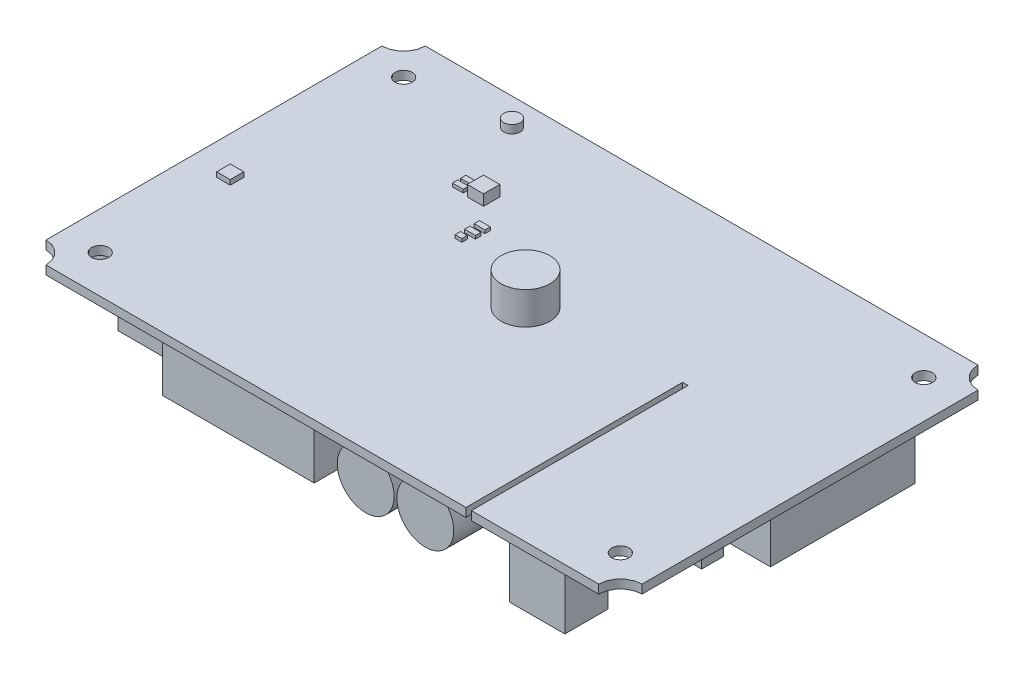
GridUp-PCB (Autodesk Fusion 360 design; units mm, degrees)
part number: 2026-09-14-08-15-55-205
Autodesk Fusion 360 part; units mm, degrees
sketch "Çizim1" plane through (0, 0, 0) normal (0, 0, 1) x (1, 0, 0)
  line L0 (0, 0) -> (110, 0)
  line L1 (110, 0) -> (110, 70)
  line L2 (110, 70) -> (0, 70)
  line L3 (0, 70) -> (0, 0)
sketch "Çizim2" plane through (0, 0, 0) normal (0, 0, 1) x (1, 0, 0)
  circle A0 centre (3.5, 3.5) radius 1.6
  circle A1 centre (106.5, 3.5) radius 1.6
  circle A2 centre (3.5, 66.5) radius 1.6
  circle A3 centre (106.5, 66.5) radius 1.6
  line L0 (81.5, -1) -> (82.5, -1)
  line L1 (82.5, -1) -> (82.5, 40)
  line L2 (82.5, 40) -> (81.5, 40)
  line L3 (81.5, 40) -> (81.5, -1)
ref_plane "WorkPlane1" through (0, 0, 1.6) normal (0, 0, 1) x (1, 0, 0)
sketch "Çizim3" plane through (0, 0, 1.6) normal (0, 0, 1) x (1, 0, 0)
  circle A0 centre (55, 37.5) radius 4.5
ref_plane "WorkPlane2" through (0, 0, 1.6) normal (0, 0, 1) x (1, 0, 0)
sketch "Çizim4" plane through (0, 0, 1.6) normal (0, 0, 1) x (1, 0, 0)
  line L0 (5.75, 29.75) -> (8.25, 29.75)
  line L1 (8.25, 29.75) -> (8.25, 32.25)
  line L2 (8.25, 32.25) -> (5.75, 32.25)
  line L3 (5.75, 32.25) -> (5.75, 29.75)
ref_plane "WorkPlane3" through (0, 0, 1.6) normal (0, 0, 1) x (1, 0, 0)
sketch "Çizim5" plane through (0, 0, 1.6) normal (0, 0, 1) x (1, 0, 0)
  circle A0 centre (25, 65) radius 1.5
ref_plane "WorkPlane4" through (0, 0, 1.6) normal (0, 0, 1) x (1, 0, 0)
sketch "Çizim6" plane through (0, 0, 1.6) normal (0, 0, 1) x (1, 0, 0)
  line L0 (37.5, 45.5) -> (39.5, 45.5)
  line L1 (39.5, 45.5) -> (39.5, 46.5)
  line L2 (39.5, 46.5) -> (37.5, 46.5)
  line L3 (37.5, 46.5) -> (37.5, 45.5)
ref_plane "WorkPlane5" through (0, 0, 1.6) normal (0, 0, 1) x (1, 0, 0)
sketch "Çizim7" plane through (0, 0, 1.6) normal (0, 0, 1) x (1, 0, 0)
  line L0 (37.5, 43.75) -> (39.5, 43.75)
  line L1 (39.5, 43.75) -> (39.5, 44.75)
  line L2 (39.5, 44.75) -> (37.5, 44.75)
  line L3 (37.5, 44.75) -> (37.5, 43.75)
ref_plane "WorkPlane6" through (0, 0, 1.6) normal (0, 0, 1) x (1, 0, 0)
sketch "Çizim8" plane through (0, 0, 1.6) normal (0, 0, 1) x (1, 0, 0)
  line L0 (37.5, 42) -> (38.75, 42)
  line L1 (38.75, 42) -> (38.75, 43)
  line L2 (38.75, 43) -> (37.5, 43)
  line L3 (37.5, 43) -> (37.5, 42)
ref_plane "WorkPlane7" through (0, 0, 1.6) normal (0, 0, 1) x (1, 0, 0)
sketch "Çizim9" plane through (0, 0, 1.6) normal (0, 0, 1) x (1, 0, 0)
  line L0 (27, 51.5) -> (29, 51.5)
  line L1 (29, 51.5) -> (29, 52.5)
  line L2 (29, 52.5) -> (27, 52.5)
  line L3 (27, 52.5) -> (27, 51.5)
ref_plane "WorkPlane8" through (0, 0, 1.6) normal (0, 0, 1) x (1, 0, 0)
sketch "Çizim10" plane through (0, 0, 1.6) normal (0, 0, 1) x (1, 0, 0)
  line L0 (27, 50) -> (29, 50)
  line L1 (29, 50) -> (29, 51)
  line L2 (29, 51) -> (27, 51)
  line L3 (27, 51) -> (27, 50)
ref_plane "WorkPlane9" through (0, 0, 1.6) normal (0, 0, 1) x (1, 0, 0)
sketch "Çizim11" plane through (0, 0, 1.6) normal (0, 0, 1) x (1, 0, 0)
  line L0 (30, 49.75) -> (33, 49.75)
  line L1 (33, 49.75) -> (33, 52.75)
  line L2 (33, 52.75) -> (30, 52.75)
  line L3 (30, 52.75) -> (30, 49.75)
ref_plane "WorkPlane10" through (0, 0, 0) normal (0, 0, 1) x (1, 0, 0)
sketch "Çizim12" plane through (0, 0, 0) normal (0, 0, 1) x (1, 0, 0)
  line L0 (6, 44.8) -> (24, 44.8)
  line L1 (24, 44.8) -> (24, 64)
  line L2 (24, 64) -> (6, 64)
  line L3 (6, 64) -> (6, 44.8)
ref_plane "WorkPlane11" through (0, 0, 0) normal (0, 0, 1) x (1, 0, 0)
sketch "Çizim13" plane through (0, 0, 0) normal (0, 0, 1) x (1, 0, 0)
  line L0 (66, 43.75) -> (99.8, 43.75)
  line L1 (99.8, 43.75) -> (99.8, 64.05)
  line L2 (99.8, 64.05) -> (66, 64.05)
  line L3 (66, 64.05) -> (66, 43.75)
ref_plane "WorkPlane12" through (0, 0, 0) normal (0, 0, 1) x (1, 0, 0)
sketch "Çizim14" plane through (0, 0, 0) normal (0, 0, 1) x (1, 0, 0)
  line L0 (88, 22.25) -> (94.1, 22.25)
  line L1 (94.1, 22.25) -> (94.1, 25)
  line L2 (94.1, 25) -> (88, 25)
  line L3 (88, 25) -> (88, 22.25)
ref_plane "WorkPlane13" through (0, 0, 0) normal (0, 0, 1) x (1, 0, 0)
sketch "Çizim15" plane through (0, 0, 0) normal (0, 0, 1) x (1, 0, 0)
  line L0 (96.5, 21.5) -> (103.5, 21.5)
  line L1 (103.5, 21.5) -> (103.5, 25.5)
  line L2 (103.5, 25.5) -> (96.5, 25.5)
  line L3 (96.5, 25.5) -> (96.5, 21.5)
ref_plane "WorkPlane14" through (0, 0, 0) normal (0, 0, 1) x (1, 0, 0)
sketch "Çizim16" plane through (0, 0, 0) normal (0, 0, 1) x (1, 0, 0)
  line L0 (92, 0.5) -> (102.25, 0.5)
  line L1 (102.25, 0.5) -> (102.25, 8.5)
  line L2 (102.25, 8.5) -> (92, 8.5)
  line L3 (92, 8.5) -> (92, 0.5)
ref_plane "WorkPlane15" through (0, 0, 0) normal (0, 0, 1) x (1, 0, 0)
sketch "Çizim17" plane through (0, 0, 0) normal (0, 0, 1) x (1, 0, 0)
  line L0 (70, 35) -> (76.5, 35)
  line L1 (76.5, 35) -> (76.5, 42)
  line L2 (76.5, 42) -> (70, 42)
  line L3 (70, 42) -> (70, 35)
ref_plane "WorkPlane16" through (0, 0, 0) normal (0, 0, 1) x (1, 0, 0)
sketch "Çizim18" plane through (0, 0, 0) normal (0, 0, 1) x (1, 0, 0)
  line L0 (76.75, 39.1) -> (81, 39.1)
  line L1 (81, 39.1) -> (81, 41.75)
  line L2 (81, 41.75) -> (76.75, 41.75)
  line L3 (76.75, 41.75) -> (76.75, 39.1)
ref_plane "WorkPlane17" through (0, 0, 0) normal (0, 0, 1) x (1, 0, 0)
sketch "Çizim19" plane through (0, 0, 0) normal (0, 0, 1) x (1, 0, 0)
  line L0 (76.75, 35.1) -> (81, 35.1)
  line L1 (81, 35.1) -> (81, 37.75)
  line L2 (81, 37.75) -> (76.75, 37.75)
  line L3 (76.75, 37.75) -> (76.75, 35.1)
ref_plane "WorkPlane18" through (0, 0, 0) normal (0, 0, 1) x (1, 0, 0)
sketch "Çizim20" plane through (0, 0, 0) normal (0, 0, 1) x (1, 0, 0)
  line L0 (75, 44.5) -> (77, 44.5)
  line L1 (77, 44.5) -> (77, 45.5)
  line L2 (77, 45.5) -> (75, 45.5)
  line L3 (75, 45.5) -> (75, 44.5)
ref_plane "WorkPlane19" through (0, 0, 0) normal (0, 0, 1) x (1, 0, 0)
sketch "Çizim21" plane through (0, 0, 0) normal (0, 0, 1) x (1, 0, 0)
  line L0 (75, 29.5) -> (77, 29.5)
  line L1 (77, 29.5) -> (77, 30.5)
  line L2 (77, 30.5) -> (75, 30.5)
  line L3 (75, 30.5) -> (75, 29.5)
ref_plane "WorkPlane20" through (0, 0, 0) normal (0, 0, 1) x (1, 0, 0)
sketch "Çizim22" plane through (0, 0, 0) normal (0, 0, 1) x (1, 0, 0)
  line L0 (75, 28) -> (77, 28)
  line L1 (77, 28) -> (77, 29)
  line L2 (77, 29) -> (75, 29)
  line L3 (75, 29) -> (75, 28)
ref_plane "WorkPlane21" through (0, 13.75, 0) normal (0, 1, 0) x (0, 0, 1)
sketch "Çizim23" plane through (0, 13.75, 0) normal (0, 1, 0) x (1, 0, 0)
  circle A0 centre (65.75, 10.75) radius 10.75
ref_plane "WorkPlane22" through (0, 0, 0) normal (0, 0, 1) x (1, 0, 0)
sketch "Çizim24" plane through (0, 0, 0) normal (0, 0, 1) x (1, 0, 0)
  line L0 (41.25, 14) -> (46.25, 14)
  line L1 (46.25, 14) -> (46.25, 20)
  line L2 (46.25, 20) -> (41.25, 20)
  line L3 (41.25, 20) -> (41.25, 14)
ref_plane "WorkPlane23" through (0, 0, 0) normal (0, 0, 1) x (1, 0, 0)
sketch "Çizim25" plane through (0, 0, 0) normal (0, 0, 1) x (1, 0, 0)
  line L0 (47.5, 15) -> (48.5, 15)
  line L1 (48.5, 15) -> (48.5, 17)
  line L2 (48.5, 17) -> (47.5, 17)
  line L3 (47.5, 17) -> (47.5, 15)
ref_plane "WorkPlane24" through (0, 0, 0) normal (0, 0, 1) x (1, 0, 0)
sketch "Çizim26" plane through (0, 0, 0) normal (0, 0, 1) x (1, 0, 0)
  line L0 (1, 6.25) -> (9, 6.25)
  line L1 (9, 6.25) -> (9, 21.5)
  line L2 (9, 21.5) -> (1, 21.5)
  line L3 (1, 21.5) -> (1, 6.25)
ref_plane "WorkPlane25" through (0, 0, 0) normal (0, 0, 1) x (1, 0, 0)
sketch "Çizim27" plane through (0, 0, 0) normal (0, 0, 1) x (1, 0, 0)
  line L0 (25, 14) -> (27, 14)
  line L1 (27, 14) -> (27, 15)
  line L2 (27, 15) -> (25, 15)
  line L3 (25, 15) -> (25, 14)
ref_plane "WorkPlane26" through (0, 0, 0) normal (0, 0, 1) x (1, 0, 0)
sketch "Çizim28" plane through (0, 0, 0) normal (0, 0, 1) x (1, 0, 0)
  line L0 (28, 14) -> (30, 14)
  line L1 (30, 14) -> (30, 15)
  line L2 (30, 15) -> (28, 15)
  line L3 (28, 15) -> (28, 14)
ref_plane "WorkPlane27" through (0, 0, 0) normal (0, 0, 1) x (1, 0, 0)
sketch "Çizim29" plane through (0, 0, 0) normal (0, 0, 1) x (1, 0, 0)
  line L0 (31, 14) -> (33, 14)
  line L1 (33, 14) -> (33, 15)
  line L2 (33, 15) -> (31, 15)
  line L3 (31, 15) -> (31, 14)
ref_plane "WorkPlane28" through (0, 0, 0) normal (0, 0, 1) x (1, 0, 0)
sketch "Çizim30" plane through (0, 0, 0) normal (0, 0, 1) x (1, 0, 0)
  line L0 (34, 14) -> (36, 14)
  line L1 (36, 14) -> (36, 15)
  line L2 (36, 15) -> (34, 15)
  line L3 (34, 15) -> (34, 14)
ref_plane "WorkPlane29" through (0, 0, 0) normal (0, 0, 1) x (1, 0, 0)
sketch "Çizim31" plane through (0, 0, 0) normal (0, 0, 1) x (1, 0, 0)
  line L0 (37, 13) -> (39, 13)
  line L1 (39, 13) -> (39, 15)
  line L2 (39, 15) -> (37, 15)
  line L3 (37, 15) -> (37, 13)
ref_plane "WorkPlane30" through (0, 0, 0) normal (0, 0, 1) x (1, 0, 0)
sketch "Çizim32" plane through (0, 0, 0) normal (0, 0, 1) x (1, 0, 0)
  line L0 (25, 0.5) -> (53, 0.5)
  line L1 (53, 0.5) -> (53, 7.5)
  line L2 (53, 7.5) -> (25, 7.5)
  line L3 (25, 7.5) -> (25, 0.5)
ref_plane "WorkPlane31" through (0, 0, 0) normal (0, 0, 1) x (1, 0, 0)
sketch "Çizim33" plane through (0, 0, 0) normal (0, 0, 1) x (1, 0, 0)
  line L0 (11, 6.25) -> (24, 6.25)
  line L1 (24, 6.25) -> (24, 11.25)
  line L2 (24, 11.25) -> (11, 11.25)
  line L3 (11, 11.25) -> (11, 6.25)
sketch "Çizim34" plane through (0, 0, 0) normal (0, 0, 1) x (1, 0, 0)
  line L0 (0, 0) -> (110, 0)
  line L1 (110, 0) -> (110, 70)
  line L2 (110, 70) -> (0, 70)
  line L3 (0, 70) -> (0, 0)
sketch "Çizim35" plane through (0, 0, 0) normal (0, 0, 1) x (1, 0, 0)
  circle A0 centre (7, 7) radius 1.6
  circle A1 centre (103, 7) radius 1.6
  circle A2 centre (7, 63) radius 1.6
  circle A3 centre (103, 63) radius 1.6
  line L0 (81.5, -1) -> (82.5, -1)
  line L1 (82.5, -1) -> (82.5, 40)
  line L2 (82.5, 40) -> (81.5, 40)
  line L3 (81.5, 40) -> (81.5, -1)
  circle A4 centre (0, 0) radius 4
  circle A5 centre (110, 0) radius 4
  circle A6 centre (0, 70) radius 4
  circle A7 centre (110, 70) radius 4
ref_plane "WorkPlane32" through (0, 0, 1.6) normal (0, 0, 1) x (1, 0, 0)
sketch "Çizim36" plane through (0, 0, 1.6) normal (0, 0, 1) x (1, 0, 0)
  circle A0 centre (55, 37.5) radius 4.5
ref_plane "WorkPlane33" through (0, 0, 1.6) normal (0, 0, 1) x (1, 0, 0)
sketch "Çizim37" plane through (0, 0, 1.6) normal (0, 0, 1) x (1, 0, 0)
  line L0 (5.75, 29.75) -> (8.25, 29.75)
  line L1 (8.25, 29.75) -> (8.25, 32.25)
  line L2 (8.25, 32.25) -> (5.75, 32.25)
  line L3 (5.75, 32.25) -> (5.75, 29.75)
ref_plane "WorkPlane34" through (0, 0, 1.6) normal (0, 0, 1) x (1, 0, 0)
sketch "Çizim38" plane through (0, 0, 1.6) normal (0, 0, 1) x (1, 0, 0)
  circle A0 centre (25, 65) radius 1.5
ref_plane "WorkPlane35" through (0, 0, 1.6) normal (0, 0, 1) x (1, 0, 0)
sketch "Çizim39" plane through (0, 0, 1.6) normal (0, 0, 1) x (1, 0, 0)
  line L0 (37.5, 45.5) -> (39.5, 45.5)
  line L1 (39.5, 45.5) -> (39.5, 46.5)
  line L2 (39.5, 46.5) -> (37.5, 46.5)
  line L3 (37.5, 46.5) -> (37.5, 45.5)
ref_plane "WorkPlane36" through (0, 0, 1.6) normal (0, 0, 1) x (1, 0, 0)
sketch "Çizim40" plane through (0, 0, 1.6) normal (0, 0, 1) x (1, 0, 0)
  line L0 (37.5, 43.75) -> (39.5, 43.75)
  line L1 (39.5, 43.75) -> (39.5, 44.75)
  line L2 (39.5, 44.75) -> (37.5, 44.75)
  line L3 (37.5, 44.75) -> (37.5, 43.75)
ref_plane "WorkPlane37" through (0, 0, 1.6) normal (0, 0, 1) x (1, 0, 0)
sketch "Çizim41" plane through (0, 0, 1.6) normal (0, 0, 1) x (1, 0, 0)
  line L0 (37.5, 42) -> (38.75, 42)
  line L1 (38.75, 42) -> (38.75, 43)
  line L2 (38.75, 43) -> (37.5, 43)
  line L3 (37.5, 43) -> (37.5, 42)
ref_plane "WorkPlane38" through (0, 0, 1.6) normal (0, 0, 1) x (1, 0, 0)
sketch "Çizim42" plane through (0, 0, 1.6) normal (0, 0, 1) x (1, 0, 0)
  line L0 (29, 51.5) -> (31, 51.5)
  line L1 (31, 51.5) -> (31, 52.5)
  line L2 (31, 52.5) -> (29, 52.5)
  line L3 (29, 52.5) -> (29, 51.5)
ref_plane "WorkPlane39" through (0, 0, 1.6) normal (0, 0, 1) x (1, 0, 0)
sketch "Çizim43" plane through (0, 0, 1.6) normal (0, 0, 1) x (1, 0, 0)
  line L0 (29, 50) -> (31, 50)
  line L1 (31, 50) -> (31, 51)
  line L2 (31, 51) -> (29, 51)
  line L3 (29, 51) -> (29, 50)
ref_plane "WorkPlane40" through (0, 0, 1.6) normal (0, 0, 1) x (1, 0, 0)
sketch "Çizim44" plane through (0, 0, 1.6) normal (0, 0, 1) x (1, 0, 0)
  line L0 (32, 49.75) -> (35, 49.75)
  line L1 (35, 49.75) -> (35, 52.75)
  line L2 (35, 52.75) -> (32, 52.75)
  line L3 (32, 52.75) -> (32, 49.75)
ref_plane "WorkPlane41" through (0, 0, 0) normal (0, 0, 1) x (1, 0, 0)
sketch "Çizim45" plane through (0, 0, 0) normal (0, 0, 1) x (1, 0, 0)
  line L0 (10, 40.8) -> (28, 40.8)
  line L1 (28, 40.8) -> (28, 60)
  line L2 (28, 60) -> (10, 60)
  line L3 (10, 60) -> (10, 40.8)
ref_plane "WorkPlane42" through (0, 0, 0) normal (0, 0, 1) x (1, 0, 0)
sketch "Çizim46" plane through (0, 0, 0) normal (0, 0, 1) x (1, 0, 0)
  line L0 (64, 43.75) -> (97.8, 43.75)
  line L1 (97.8, 43.75) -> (97.8, 64.05)
  line L2 (97.8, 64.05) -> (64, 64.05)
  line L3 (64, 64.05) -> (64, 43.75)
ref_plane "WorkPlane43" through (0, 0, 0) normal (0, 0, 1) x (1, 0, 0)
sketch "Çizim47" plane through (0, 0, 0) normal (0, 0, 1) x (1, 0, 0)
  line L0 (88, 22.25) -> (94.1, 22.25)
  line L1 (94.1, 22.25) -> (94.1, 25)
  line L2 (94.1, 25) -> (88, 25)
  line L3 (88, 25) -> (88, 22.25)
ref_plane "WorkPlane44" through (0, 0, 0) normal (0, 0, 1) x (1, 0, 0)
sketch "Çizim48" plane through (0, 0, 0) normal (0, 0, 1) x (1, 0, 0)
  line L0 (96.5, 21.5) -> (103.5, 21.5)
  line L1 (103.5, 21.5) -> (103.5, 25.5)
  line L2 (103.5, 25.5) -> (96.5, 25.5)
  line L3 (96.5, 25.5) -> (96.5, 21.5)
ref_plane "WorkPlane45" through (0, 0, 0) normal (0, 0, 1) x (1, 0, 0)
sketch "Çizim49" plane through (0, 0, 0) normal (0, 0, 1) x (1, 0, 0)
  line L0 (89, 0.5) -> (99.25, 0.5)
  line L1 (99.25, 0.5) -> (99.25, 8.5)
  line L2 (99.25, 8.5) -> (89, 8.5)
  line L3 (89, 8.5) -> (89, 0.5)
ref_plane "WorkPlane46" through (0, 0, 0) normal (0, 0, 1) x (1, 0, 0)
sketch "Çizim50" plane through (0, 0, 0) normal (0, 0, 1) x (1, 0, 0)
  line L0 (70, 35) -> (76.5, 35)
  line L1 (76.5, 35) -> (76.5, 42)
  line L2 (76.5, 42) -> (70, 42)
  line L3 (70, 42) -> (70, 35)
ref_plane "WorkPlane47" through (0, 0, 0) normal (0, 0, 1) x (1, 0, 0)
sketch "Çizim51" plane through (0, 0, 0) normal (0, 0, 1) x (1, 0, 0)
  line L0 (76.75, 39.1) -> (81, 39.1)
  line L1 (81, 39.1) -> (81, 41.75)
  line L2 (81, 41.75) -> (76.75, 41.75)
  line L3 (76.75, 41.75) -> (76.75, 39.1)
ref_plane "WorkPlane48" through (0, 0, 0) normal (0, 0, 1) x (1, 0, 0)
sketch "Çizim52" plane through (0, 0, 0) normal (0, 0, 1) x (1, 0, 0)
  line L0 (76.75, 35.1) -> (81, 35.1)
  line L1 (81, 35.1) -> (81, 37.75)
  line L2 (81, 37.75) -> (76.75, 37.75)
  line L3 (76.75, 37.75) -> (76.75, 35.1)
ref_plane "WorkPlane49" through (0, 0, 0) normal (0, 0, 1) x (1, 0, 0)
sketch "Çizim53" plane through (0, 0, 0) normal (0, 0, 1) x (1, 0, 0)
  line L0 (60.5, 44.5) -> (62.5, 44.5)
  line L1 (62.5, 44.5) -> (62.5, 45.5)
  line L2 (62.5, 45.5) -> (60.5, 45.5)
  line L3 (60.5, 45.5) -> (60.5, 44.5)
ref_plane "WorkPlane50" through (0, 0, 0) normal (0, 0, 1) x (1, 0, 0)
sketch "Çizim54" plane through (0, 0, 0) normal (0, 0, 1) x (1, 0, 0)
  line L0 (75, 29.5) -> (77, 29.5)
  line L1 (77, 29.5) -> (77, 30.5)
  line L2 (77, 30.5) -> (75, 30.5)
  line L3 (75, 30.5) -> (75, 29.5)
ref_plane "WorkPlane51" through (0, 0, 0) normal (0, 0, 1) x (1, 0, 0)
sketch "Çizim55" plane through (0, 0, 0) normal (0, 0, 1) x (1, 0, 0)
  line L0 (75, 28) -> (77, 28)
  line L1 (77, 28) -> (77, 29)
  line L2 (77, 29) -> (75, 29)
  line L3 (75, 29) -> (75, 28)
ref_plane "WorkPlane52" through (0, 13.75, 0) normal (0, 1, 0) x (0, 0, 1)
sketch "Çizim56" plane through (0, 13.75, 0) normal (0, 1, 0) x (1, 0, 0)
  circle A0 centre (65.75, 10.75) radius 10.75
ref_plane "WorkPlane53" through (0, 0, 0) normal (0, 0, 1) x (1, 0, 0)
sketch "Çizim57" plane through (0, 0, 0) normal (0, 0, 1) x (1, 0, 0)
  line L0 (41.25, 14) -> (46.25, 14)
  line L1 (46.25, 14) -> (46.25, 20)
  line L2 (46.25, 20) -> (41.25, 20)
  line L3 (41.25, 20) -> (41.25, 14)
ref_plane "WorkPlane54" through (0, 0, 0) normal (0, 0, 1) x (1, 0, 0)
sketch "Çizim58" plane through (0, 0, 0) normal (0, 0, 1) x (1, 0, 0)
  line L0 (47.5, 15) -> (48.5, 15)
  line L1 (48.5, 15) -> (48.5, 17)
  line L2 (48.5, 17) -> (47.5, 17)
  line L3 (47.5, 17) -> (47.5, 15)
ref_plane "WorkPlane55" through (0, 0, 0) normal (0, 0, 1) x (1, 0, 0)
sketch "Çizim59" plane through (0, 0, 0) normal (0, 0, 1) x (1, 0, 0)
  line L0 (1, 11) -> (9, 11)
  line L1 (9, 11) -> (9, 26.25)
  line L2 (9, 26.25) -> (1, 26.25)
  line L3 (1, 26.25) -> (1, 11)
ref_plane "WorkPlane56" through (0, 0, 0) normal (0, 0, 1) x (1, 0, 0)
sketch "Çizim60" plane through (0, 0, 0) normal (0, 0, 1) x (1, 0, 0)
  line L0 (25, 14) -> (27, 14)
  line L1 (27, 14) -> (27, 15)
  line L2 (27, 15) -> (25, 15)
  line L3 (25, 15) -> (25, 14)
ref_plane "WorkPlane57" through (0, 0, 0) normal (0, 0, 1) x (1, 0, 0)
sketch "Çizim61" plane through (0, 0, 0) normal (0, 0, 1) x (1, 0, 0)
  line L0 (28, 14) -> (30, 14)
  line L1 (30, 14) -> (30, 15)
  line L2 (30, 15) -> (28, 15)
  line L3 (28, 15) -> (28, 14)
ref_plane "WorkPlane58" through (0, 0, 0) normal (0, 0, 1) x (1, 0, 0)
sketch "Çizim62" plane through (0, 0, 0) normal (0, 0, 1) x (1, 0, 0)
  line L0 (31, 14) -> (33, 14)
  line L1 (33, 14) -> (33, 15)
  line L2 (33, 15) -> (31, 15)
  line L3 (31, 15) -> (31, 14)
ref_plane "WorkPlane59" through (0, 0, 0) normal (0, 0, 1) x (1, 0, 0)
sketch "Çizim63" plane through (0, 0, 0) normal (0, 0, 1) x (1, 0, 0)
  line L0 (34, 14) -> (36, 14)
  line L1 (36, 14) -> (36, 15)
  line L2 (36, 15) -> (34, 15)
  line L3 (34, 15) -> (34, 14)
ref_plane "WorkPlane60" through (0, 0, 0) normal (0, 0, 1) x (1, 0, 0)
sketch "Çizim64" plane through (0, 0, 0) normal (0, 0, 1) x (1, 0, 0)
  line L0 (37, 13) -> (39, 13)
  line L1 (39, 13) -> (39, 15)
  line L2 (39, 15) -> (37, 15)
  line L3 (37, 15) -> (37, 13)
ref_plane "WorkPlane61" through (0, 0, 0) normal (0, 0, 1) x (1, 0, 0)
sketch "Çizim65" plane through (0, 0, 0) normal (0, 0, 1) x (1, 0, 0)
  line L0 (25, 0.5) -> (53, 0.5)
  line L1 (53, 0.5) -> (53, 7.5)
  line L2 (53, 7.5) -> (25, 7.5)
  line L3 (25, 7.5) -> (25, 0.5)
ref_plane "WorkPlane62" through (0, 0, 0) normal (0, 0, 1) x (1, 0, 0)
sketch "Çizim66" plane through (0, 0, 0) normal (0, 0, 1) x (1, 0, 0)
  line L0 (11, 6.25) -> (24, 6.25)
  line L1 (24, 6.25) -> (24, 11.25)
  line L2 (24, 11.25) -> (11, 11.25)
  line L3 (11, 11.25) -> (11, 6.25)
sketch "Çizim67" plane through (0, 0, 0) normal (0, 0, 1) x (1, 0, 0)
  line L0 (0, 0) -> (110, 0)
  line L1 (110, 0) -> (110, 70)
  line L2 (110, 70) -> (0, 70)
  line L3 (0, 70) -> (0, 0)
extrude "Ekstrüzyon67" add sketch "Çizim67" along normal blind 1.6 makes body 1
fillet "Radyus3" radius 2 4 edges at (0, 70, 0.8) (110, 70, 0.8) (110, 0, 0.8) (0, 0, 0.8) on bodies 1
sketch "Çizim68" plane through (0, 0, 0) normal (0, 0, 1) x (1, 0, 0)
  circle A0 centre (7, 7) radius 1.6
  circle A1 centre (103, 7) radius 1.6
  circle A2 centre (7, 63) radius 1.6
  circle A3 centre (103, 63) radius 1.6
  line L0 (81.5, -1) -> (82.5, -1)
  line L1 (82.5, -1) -> (82.5, 40)
  line L2 (82.5, 40) -> (81.5, 40)
  line L3 (81.5, 40) -> (81.5, -1)
  circle A4 centre (0, 0) radius 4
  circle A5 centre (110, 0) radius 4
  circle A6 centre (0, 70) radius 4
  circle A7 centre (110, 70) radius 4
extrude "Ekstrüzyon68" cut sketch "Çizim68" along normal mid plane 10 bodies 1
ref_plane "WorkPlane63" through (0, 0, 1.6) normal (0, 0, 1) x (1, 0, 0)
sketch "Çizim69" plane through (0, 0, 1.6) normal (0, 0, 1) x (1, 0, 0)
  circle A0 centre (55, 37.5) radius 4.5
extrude "Ekstrüzyon69" add sketch "Çizim69" along normal blind 6 separate body makes body 2
ref_plane "WorkPlane64" through (0, 0, 1.6) normal (0, 0, 1) x (1, 0, 0)
sketch "Çizim70" plane through (0, 0, 1.6) normal (0, 0, 1) x (1, 0, 0)
  line L0 (5.75, 29.75) -> (8.25, 29.75)
  line L1 (8.25, 29.75) -> (8.25, 32.25)
  line L2 (8.25, 32.25) -> (5.75, 32.25)
  line L3 (5.75, 32.25) -> (5.75, 29.75)
extrude "Ekstrüzyon70" add sketch "Çizim70" along normal blind 0.9 separate body makes body 3
ref_plane "WorkPlane65" through (0, 0, 1.6) normal (0, 0, 1) x (1, 0, 0)
sketch "Çizim71" plane through (0, 0, 1.6) normal (0, 0, 1) x (1, 0, 0)
  circle A0 centre (25, 65) radius 1.5
extrude "Ekstrüzyon71" add sketch "Çizim71" along normal blind 1.5 separate body makes body 4
ref_plane "WorkPlane66" through (0, 0, 1.6) normal (0, 0, 1) x (1, 0, 0)
sketch "Çizim72" plane through (0, 0, 1.6) normal (0, 0, 1) x (1, 0, 0)
  line L0 (37.5, 45.5) -> (39.5, 45.5)
  line L1 (39.5, 45.5) -> (39.5, 46.5)
  line L2 (39.5, 46.5) -> (37.5, 46.5)
  line L3 (37.5, 46.5) -> (37.5, 45.5)
extrude "Ekstrüzyon72" add sketch "Çizim72" along normal blind 0.6 separate body makes body 5
ref_plane "WorkPlane67" through (0, 0, 1.6) normal (0, 0, 1) x (1, 0, 0)
sketch "Çizim73" plane through (0, 0, 1.6) normal (0, 0, 1) x (1, 0, 0)
  line L0 (37.5, 43.75) -> (39.5, 43.75)
  line L1 (39.5, 43.75) -> (39.5, 44.75)
  line L2 (39.5, 44.75) -> (37.5, 44.75)
  line L3 (37.5, 44.75) -> (37.5, 43.75)
extrude "Ekstrüzyon73" add sketch "Çizim73" along normal blind 0.6 separate body makes body 6
ref_plane "WorkPlane68" through (0, 0, 1.6) normal (0, 0, 1) x (1, 0, 0)
sketch "Çizim74" plane through (0, 0, 1.6) normal (0, 0, 1) x (1, 0, 0)
  line L0 (37.5, 42) -> (38.75, 42)
  line L1 (38.75, 42) -> (38.75, 43)
  line L2 (38.75, 43) -> (37.5, 43)
  line L3 (37.5, 43) -> (37.5, 42)
extrude "Ekstrüzyon74" add sketch "Çizim74" along normal blind 0.6 separate body makes body 7
ref_plane "WorkPlane69" through (0, 0, 1.6) normal (0, 0, 1) x (1, 0, 0)
sketch "Çizim75" plane through (0, 0, 1.6) normal (0, 0, 1) x (1, 0, 0)
  line L0 (29, 51.5) -> (31, 51.5)
  line L1 (31, 51.5) -> (31, 52.5)
  line L2 (31, 52.5) -> (29, 52.5)
  line L3 (29, 52.5) -> (29, 51.5)
extrude "Ekstrüzyon75" add sketch "Çizim75" along normal blind 0.6 separate body makes body 8
ref_plane "WorkPlane70" through (0, 0, 1.6) normal (0, 0, 1) x (1, 0, 0)
sketch "Çizim76" plane through (0, 0, 1.6) normal (0, 0, 1) x (1, 0, 0)
  line L0 (29, 50) -> (31, 50)
  line L1 (31, 50) -> (31, 51)
  line L2 (31, 51) -> (29, 51)
  line L3 (29, 51) -> (29, 50)
extrude "Ekstrüzyon76" add sketch "Çizim76" along normal blind 0.6 separate body makes body 9
ref_plane "WorkPlane71" through (0, 0, 1.6) normal (0, 0, 1) x (1, 0, 0)
sketch "Çizim77" plane through (0, 0, 1.6) normal (0, 0, 1) x (1, 0, 0)
  line L0 (32, 49.75) -> (35, 49.75)
  line L1 (35, 49.75) -> (35, 52.75)
  line L2 (35, 52.75) -> (32, 52.75)
  line L3 (32, 52.75) -> (32, 49.75)
extrude "Ekstrüzyon77" add sketch "Çizim77" along normal blind 2 separate body makes body 10
ref_plane "WorkPlane72" through (0, 0, 0) normal (0, 0, 1) x (1, 0, 0)
sketch "Çizim78" plane through (0, 0, 0) normal (0, 0, 1) x (1, 0, 0)
  line L0 (10, 40.8) -> (28, 40.8)
  line L1 (28, 40.8) -> (28, 60)
  line L2 (28, 60) -> (10, 60)
  line L3 (10, 60) -> (10, 40.8)
extrude "Ekstrüzyon78" add sketch "Çizim78" against normal blind 3.2 separate body makes body 11
ref_plane "WorkPlane73" through (0, 0, 0) normal (0, 0, 1) x (1, 0, 0)
sketch "Çizim79" plane through (0, 0, 0) normal (0, 0, 1) x (1, 0, 0)
  line L0 (64, 42) -> (95.7, 42)
  line L1 (95.7, 42) -> (95.7, 68.7)
  line L2 (95.7, 68.7) -> (64, 68.7)
  line L3 (64, 68.7) -> (64, 42)
extrude "Ekstrüzyon79" add sketch "Çizim79" against normal blind 21.8 separate body makes body 12
ref_plane "WorkPlane74" through (0, 0, 0) normal (0, 0, 1) x (1, 0, 0)
sketch "Çizim80" plane through (0, 0, 0) normal (0, 0, 1) x (1, 0, 0)
  line L0 (88, 22.25) -> (94.1, 22.25)
  line L1 (94.1, 22.25) -> (94.1, 25)
  line L2 (94.1, 25) -> (88, 25)
  line L3 (88, 25) -> (88, 22.25)
extrude "Ekstrüzyon80" add sketch "Çizim80" against normal blind 2.6 separate body makes body 13
ref_plane "WorkPlane75" through (0, 0, 0) normal (0, 0, 1) x (1, 0, 0)
sketch "Çizim81" plane through (0, 0, 0) normal (0, 0, 1) x (1, 0, 0)
  line L0 (96.5, 21.5) -> (103.5, 21.5)
  line L1 (103.5, 21.5) -> (103.5, 25.5)
  line L2 (103.5, 25.5) -> (96.5, 25.5)
  line L3 (96.5, 25.5) -> (96.5, 21.5)
extrude "Ekstrüzyon81" add sketch "Çizim81" against normal blind 8 separate body makes body 14
ref_plane "WorkPlane76" through (0, 0, 0) normal (0, 0, 1) x (1, 0, 0)
sketch "Çizim82" plane through (0, 0, 0) normal (0, 0, 1) x (1, 0, 0)
  line L0 (89, 0.5) -> (99.25, 0.5)
  line L1 (99.25, 0.5) -> (99.25, 8.5)
  line L2 (99.25, 8.5) -> (89, 8.5)
  line L3 (89, 8.5) -> (89, 0.5)
extrude "Ekstrüzyon82" add sketch "Çizim82" against normal blind 10 separate body makes body 15
ref_plane "WorkPlane77" through (0, 0, 0) normal (0, 0, 1) x (1, 0, 0)
sketch "Çizim83" plane through (0, 0, 0) normal (0, 0, 1) x (1, 0, 0)
  line L0 (70, 34) -> (76.5, 34)
  line L1 (76.5, 34) -> (76.5, 41)
  line L2 (76.5, 41) -> (70, 41)
  line L3 (70, 41) -> (70, 34)
extrude "Ekstrüzyon83" add sketch "Çizim83" against normal blind 1.7 separate body makes body 16
ref_plane "WorkPlane78" through (0, 0, 0) normal (0, 0, 1) x (1, 0, 0)
sketch "Çizim84" plane through (0, 0, 0) normal (0, 0, 1) x (1, 0, 0)
  line L0 (76.75, 39) -> (81, 39)
  line L1 (81, 39) -> (81, 41.65)
  line L2 (81, 41.65) -> (76.75, 41.65)
  line L3 (76.75, 41.65) -> (76.75, 39)
extrude "Ekstrüzyon84" add sketch "Çizim84" against normal blind 1.5 separate body makes body 17
ref_plane "WorkPlane79" through (0, 0, 0) normal (0, 0, 1) x (1, 0, 0)
sketch "Çizim85" plane through (0, 0, 0) normal (0, 0, 1) x (1, 0, 0)
  line L0 (76.75, 35) -> (81, 35)
  line L1 (81, 35) -> (81, 37.65)
  line L2 (81, 37.65) -> (76.75, 37.65)
  line L3 (76.75, 37.65) -> (76.75, 35)
extrude "Ekstrüzyon85" add sketch "Çizim85" against normal blind 1.5 separate body makes body 18
ref_plane "WorkPlane80" through (0, 0, 0) normal (0, 0, 1) x (1, 0, 0)
sketch "Çizim86" plane through (0, 0, 0) normal (0, 0, 1) x (1, 0, 0)
  line L0 (60.5, 44.5) -> (62.5, 44.5)
  line L1 (62.5, 44.5) -> (62.5, 45.5)
  line L2 (62.5, 45.5) -> (60.5, 45.5)
  line L3 (60.5, 45.5) -> (60.5, 44.5)
extrude "Ekstrüzyon86" add sketch "Çizim86" against normal blind 0.6 separate body makes body 19
ref_plane "WorkPlane81" through (0, 0, 0) normal (0, 0, 1) x (1, 0, 0)
sketch "Çizim87" plane through (0, 0, 0) normal (0, 0, 1) x (1, 0, 0)
  line L0 (77.5, 29.5) -> (79.5, 29.5)
  line L1 (79.5, 29.5) -> (79.5, 30.5)
  line L2 (79.5, 30.5) -> (77.5, 30.5)
  line L3 (77.5, 30.5) -> (77.5, 29.5)
extrude "Ekstrüzyon87" add sketch "Çizim87" against normal blind 0.6 separate body makes body 20
ref_plane "WorkPlane82" through (0, 0, 0) normal (0, 0, 1) x (1, 0, 0)
sketch "Çizim88" plane through (0, 0, 0) normal (0, 0, 1) x (1, 0, 0)
  line L0 (77.5, 28) -> (79.5, 28)
  line L1 (79.5, 28) -> (79.5, 29)
  line L2 (79.5, 29) -> (77.5, 29)
  line L3 (77.5, 29) -> (77.5, 28)
extrude "Ekstrüzyon88" add sketch "Çizim88" against normal blind 0.6 separate body makes body 21
ref_plane "WorkPlane83" through (0, 0, 0) normal (0, 0, 1) x (1, 0, 0)
sketch "Çizim89" plane through (0, 0, 0) normal (0, 0, 1) x (1, 0, 0)
  line L0 (55, 36) -> (57.5, 36)
  line L1 (57.5, 36) -> (57.5, 38)
  line L2 (57.5, 38) -> (55, 38)
  line L3 (55, 38) -> (55, 36)
extrude "Ekstrüzyon89" add sketch "Çizim89" against normal blind 1 separate body makes body 22
ref_plane "WorkPlane84" through (0, 0, 0) normal (0, 0, 1) x (1, 0, 0)
sketch "Çizim90" plane through (0, 0, 0) normal (0, 0, 1) x (1, 0, 0)
  line L0 (59, 35.5) -> (62, 35.5)
  line L1 (62, 35.5) -> (62, 38.5)
  line L2 (62, 38.5) -> (59, 38.5)
  line L3 (59, 38.5) -> (59, 35.5)
extrude "Ekstrüzyon90" add sketch "Çizim90" against normal blind 1.5 separate body makes body 23
ref_plane "WorkPlane85" through (0, 0, 0) normal (0, 0, 1) x (1, 0, 0)
sketch "Çizim91" plane through (0, 0, 0) normal (0, 0, 1) x (1, 0, 0)
  line L0 (52, 28) -> (54, 28)
  line L1 (54, 28) -> (54, 29)
  line L2 (54, 29) -> (52, 29)
  line L3 (52, 29) -> (52, 28)
extrude "Ekstrüzyon91" add sketch "Çizim91" against normal blind 0.6 separate body makes body 24
ref_plane "WorkPlane86" through (0, 0, 0) normal (0, 0, 1) x (1, 0, 0)
sketch "Çizim92" plane through (0, 0, 0) normal (0, 0, 1) x (1, 0, 0)
  line L0 (52, 30.5) -> (54, 30.5)
  line L1 (54, 30.5) -> (54, 31.5)
  line L2 (54, 31.5) -> (52, 31.5)
  line L3 (52, 31.5) -> (52, 30.5)
extrude "Ekstrüzyon92" add sketch "Çizim92" against normal blind 0.6 separate body makes body 25
ref_plane "WorkPlane87" through (0, 17.75, 0) normal (0, 1, 0) x (0, 0, 1)
sketch "Çizim93" plane through (0, 17.75, 0) normal (0, 1, 0) x (1, 0, 0)
  circle A0 centre (61, 5.25) radius 5.25
extrude "Ekstrüzyon93" add sketch "Çizim93" along normal mid plane 31.5 separate body makes body 26
sketch "Çizim94" plane through (0, 17.75, 0) normal (0, 1, 0) x (1, 0, 0)
  circle A0 centre (72, 5.25) radius 5.25
extrude "Ekstrüzyon94" add sketch "Çizim94" along normal mid plane 31.5 separate body makes body 27
ref_plane "WorkPlane88" through (0, 0, 0) normal (0, 0, 1) x (1, 0, 0)
sketch "Çizim95" plane through (0, 0, 0) normal (0, 0, 1) x (1, 0, 0)
  line L0 (41.25, 14) -> (46.25, 14)
  line L1 (46.25, 14) -> (46.25, 20)
  line L2 (46.25, 20) -> (41.25, 20)
  line L3 (41.25, 20) -> (41.25, 14)
extrude "Ekstrüzyon95" add sketch "Çizim95" against normal blind 1.5 separate body makes body 28
ref_plane "WorkPlane89" through (0, 0, 0) normal (0, 0, 1) x (1, 0, 0)
sketch "Çizim96" plane through (0, 0, 0) normal (0, 0, 1) x (1, 0, 0)
  line L0 (47.5, 15) -> (48.5, 15)
  line L1 (48.5, 15) -> (48.5, 17)
  line L2 (48.5, 17) -> (47.5, 17)
  line L3 (47.5, 17) -> (47.5, 15)
extrude "Ekstrüzyon96" add sketch "Çizim96" against normal blind 0.6 separate body makes body 29
ref_plane "WorkPlane90" through (0, 0, 0) normal (0, 0, 1) x (1, 0, 0)
sketch "Çizim97" plane through (0, 0, 0) normal (0, 0, 1) x (1, 0, 0)
  line L0 (1, 11) -> (9, 11)
  line L1 (9, 11) -> (9, 26.25)
  line L2 (9, 26.25) -> (1, 26.25)
  line L3 (1, 26.25) -> (1, 11)
extrude "Ekstrüzyon97" add sketch "Çizim97" against normal blind 10 separate body makes body 30
ref_plane "WorkPlane91" through (0, 0, 0) normal (0, 0, 1) x (1, 0, 0)
sketch "Çizim98" plane through (0, 0, 0) normal (0, 0, 1) x (1, 0, 0)
  line L0 (25, 14) -> (27, 14)
  line L1 (27, 14) -> (27, 15)
  line L2 (27, 15) -> (25, 15)
  line L3 (25, 15) -> (25, 14)
extrude "Ekstrüzyon98" add sketch "Çizim98" against normal blind 0.6 separate body makes body 31
ref_plane "WorkPlane92" through (0, 0, 0) normal (0, 0, 1) x (1, 0, 0)
sketch "Çizim99" plane through (0, 0, 0) normal (0, 0, 1) x (1, 0, 0)
  line L0 (28, 14) -> (30, 14)
  line L1 (30, 14) -> (30, 15)
  line L2 (30, 15) -> (28, 15)
  line L3 (28, 15) -> (28, 14)
extrude "Ekstrüzyon99" add sketch "Çizim99" against normal blind 0.6 separate body makes body 32
ref_plane "WorkPlane93" through (0, 0, 0) normal (0, 0, 1) x (1, 0, 0)
sketch "Çizim100" plane through (0, 0, 0) normal (0, 0, 1) x (1, 0, 0)
  line L0 (31, 14) -> (33, 14)
  line L1 (33, 14) -> (33, 15)
  line L2 (33, 15) -> (31, 15)
  line L3 (31, 15) -> (31, 14)
extrude "Ekstrüzyon100" add sketch "Çizim100" against normal blind 0.6 separate body makes body 33
ref_plane "WorkPlane94" through (0, 0, 0) normal (0, 0, 1) x (1, 0, 0)
sketch "Çizim101" plane through (0, 0, 0) normal (0, 0, 1) x (1, 0, 0)
  line L0 (34, 14) -> (36, 14)
  line L1 (36, 14) -> (36, 15)
  line L2 (36, 15) -> (34, 15)
  line L3 (34, 15) -> (34, 14)
extrude "Ekstrüzyon101" add sketch "Çizim101" against normal blind 0.6 separate body makes body 34
ref_plane "WorkPlane95" through (0, 0, 0) normal (0, 0, 1) x (1, 0, 0)
sketch "Çizim102" plane through (0, 0, 0) normal (0, 0, 1) x (1, 0, 0)
  line L0 (37, 13) -> (39, 13)
  line L1 (39, 13) -> (39, 15)
  line L2 (39, 15) -> (37, 15)
  line L3 (37, 15) -> (37, 13)
extrude "Ekstrüzyon102" add sketch "Çizim102" against normal blind 0.6 separate body makes body 35
ref_plane "WorkPlane96" through (0, 0, 0) normal (0, 0, 1) x (1, 0, 0)
sketch "Çizim103" plane through (0, 0, 0) normal (0, 0, 1) x (1, 0, 0)
  line L0 (25, 0.5) -> (53, 0.5)
  line L1 (53, 0.5) -> (53, 7.5)
  line L2 (53, 7.5) -> (25, 7.5)
  line L3 (25, 7.5) -> (25, 0.5)
extrude "Ekstrüzyon103" add sketch "Çizim103" against normal blind 9 separate body makes body 36
ref_plane "WorkPlane97" through (0, 0, 0) normal (0, 0, 1) x (1, 0, 0)
sketch "Çizim104" plane through (0, 0, 0) normal (0, 0, 1) x (1, 0, 0)
  line L0 (11, 6.25) -> (24, 6.25)
  line L1 (24, 6.25) -> (24, 11.25)
  line L2 (24, 11.25) -> (11, 11.25)
  line L3 (11, 11.25) -> (11, 6.25)
extrude "Ekstrüzyon104" add sketch "Çizim104" against normal blind 8.5 separate body makes body 37
equation "d305 = -( 3.2 mm )"
equation "d309 = -( 21.8 mm )"
equation "d313 = -( 2.6 mm )"
equation "d317 = -( 8 mm )"
equation "d321 = -( 10 mm )"
equation "d325 = -( 1.7 mm )"
equation "d329 = -( 1.5 mm )"
equation "d333 = -( 1.5 mm )"
equation "d337 = -( 0.6 mm )"
equation "d341 = -( 0.6 mm )"
equation "d345 = -( 0.6 mm )"
equation "d349 = -( 1 mm )"
equation "d353 = -( 1.5 mm )"
equation "d357 = -( 0.6 mm )"
equation "d361 = -( 0.6 mm )"
equation "d371 = -( 1.5 mm )"
equation "d375 = -( 0.6 mm )"
equation "d379 = -( 10 mm )"
equation "d383 = -( 0.6 mm )"
equation "d387 = -( 0.6 mm )"
equation "d391 = -( 0.6 mm )"
equation "d395 = -( 0.6 mm )"
equation "d399 = -( 0.6 mm )"
equation "d403 = -( 9 mm )"
equation "d407 = -( 8.5 mm )"
named bodies: "PCB", "MLX90640", "SHT31", "LED", "R_pullup1", "R_pullup2", "C_100n", "EN_RC1", "EN_RC2", "Reset", "ESP32-S3-WROOM-1U", "RAC05-05SK", "F1", "MOV", "Klemens 230V", "LDO SOT-223", "D1", "D2", "R_sarj", "Bolucu1", "Bolucu2", "Boost U7", "L_boost", "R_bal1", "R_bal2", "Superkap1", "Superkap2", "MAX3485", "R120", "Klemens RS-485", "R_burden1", "R_burden2", "R_burden3", "R_burden4", "R_bias", "Klemens CT", "Genisleme 2x5"
